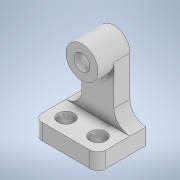
# Autodesk Inventor part: 7.1 Part 5
Saved by Autodesk Inventor 2020 (Build 240168000, 168)
## iProperties
Created: 2020-03-12
Part Number: 7.1 Part 5
Material: Generic
Document SubType Name: Modeling
Designer: cks4a449
Density: 1 g/cm^3
Appearance: Default
Author: cks4a449
Autodesk Inventor part; units mm, degrees
ref_plane "YZ Plane" through (0, 0, 0) normal (1, 0, 0) x (0, 1, 0)
ref_plane "XZ Plane" through (0, 0, 0) normal (0, 1, 0) x (-1, 0, 0)
ref_plane "XY Plane" through (0, 0, 0) normal (0, 0, 1) x (1, 0, 0)
sketch "Sketch1" plane through (0, 0, 0) normal (0, 1, 0) x (-1, 0, 0)
  line L0 (6.35, 0) -> (44.45, 0)
  line L1 (50.8, -6.35) -> (50.8, -38.1)
  line L2 (50.8, -38.1) -> (0, -38.1)
  line L3 (0, -38.1) -> (0, -6.35)
  arc A0 (50.8, -6.35) -> (44.45, 0) centre (44.45, -6.35) ccw
  arc A1 (6.35, 0) -> (0, -6.35) centre (6.35, -6.35) ccw
  point P0 (0, 0)
  point P1 (50.8, 0)
  dimension "d0" = 50.8
  dimension "d1" = 38.1
  dimension "d2" = 6.35
  dimension "d3" = 6.35
  constraints: 8 end point, 4 point on circle, 4 point on line, 4 tangent, 2 centre point, 2 parallel, 1 horizontal, 1 perpendicular
  measures "d0" distance of L1.end L2.end
  measures "d1" distance of point (50.8, 0) L1.end
  measures "d2" radius of A0
  measures "d3" radius of A1
extrude "Extrusion1" add sketch "Sketch1" along normal blind 12.7
sketch "Sketch2" plane through (0, 0, -38.1) normal (0, 0, -1) x (-1, 0, 0)
  circle A0 centre (25.4, 57.15) radius 6.35
  circle A1 centre (25.4, 57.15) radius 12.7
  line L0 (38.1, 25.4) -> (38.1, 57.15)
  line L1 (12.7, 57.15) -> (12.7, 25.4)
  line L2 (0, 12.7) -> (50.8, 12.7) projected
  line L3 (6.35, 12.7) -> (0, 12.7) projected
  arc A2 (0, 12.7) -> (12.7, 25.4) centre (0, 25.4) ccw
  arc A3 (38.1, 25.4) -> (50.8, 12.7) centre (50.8, 25.4) ccw
  point P0 (0, 0)
  point P1 (25.4, 12.7)
  dimension "d6" = 12.7
  dimension "d7" = 25.4
  dimension "d12" = 44.45
  constraints: 7 point on circle, 6 tangent, 4 centre point, 4 end point, 1 coincident, 1 midpoint, 1 parallel
  measures "d6" diameter of A0
  measures "d7" diameter of A1
  measures "d12" distance from line of L2 A0.centre
extrude "Extrusion2" add sketch "Sketch2" against normal blind 12.7 contours L0 A3 L2 A2 L1 A1
extrude "Extrusion3" add sketch "Sketch2" against normal blind 25.4 contours A1
sketch "Sketch3" plane through (0, 12.7, 0) normal (0, 1, 0) x (1, 0, 0)
  circle A0 centre (-38.1, 12.7) radius 6.35
  circle A1 centre (-12.7, 12.7) radius 6.35
  line L0 (-44.45, 0) -> (-6.35, 0) projected
  line L1 (0, 6.35) -> (0, 25.4) projected
  line L2 (-50.8, 25.4) -> (-50.8, 6.35) projected
  point P0 (0, 0)
  dimension "d17" = 12.7
  dimension "d18" = 12.7
  dimension "d19" = 12.7
  dimension "d20" = 12.7
  dimension "d21" = 12.7
  dimension "d22" = 12.7
  constraints: 2 centre point
  measures "d17" diameter of A0
  measures "d18" diameter of A1
  measures "d19" distance from line of L0 A1.centre
  measures "d20" distance from line of L1 A1.centre
  measures "d21" distance from line of L0 A0.centre
  measures "d22" distance from line of L2 A0.centre
extrude "Extrusion4" cut sketch "Sketch3" against normal through all
body "Solid1"
